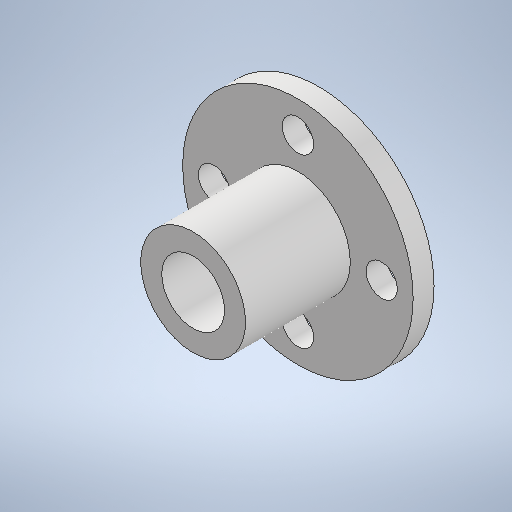
# Autodesk Inventor part: 驱动轮法兰
Saved by Autodesk Inventor 2025.1 (Build 291241000, 241)
## iProperties
Created: 2025-08-26
Part Number: 驱动轮法兰
Material: 常规
Document SubType Name: Modeling
Designer: Piw
Density: 1 g/cm^3
Appearance: 默认
Author: Piw
Autodesk Inventor part; units mm, degrees
ref_plane "YZ Plane" through (0, 0, 0) normal (1, 0, 0) x (0, 1, 0)
ref_plane "XZ Plane" through (0, 0, 0) normal (0, 1, 0) x (-1, 0, 0)
ref_plane "XY Plane" through (0, 0, 0) normal (0, 0, 1) x (1, 0, 0)
sketch "草图1" plane through (0, 0, 0) normal (0, 0, 1) x (1, 0, 0)
  circle A0 centre (0, 0) radius 11
  circle A1 centre (0, 0) radius 3
  dimension "d0" = 22
  dimension "d1" = 6
  constraints: 2 centre point, 2 coincident
  measures "d0" diameter of A0
  measures "d1" diameter of A1
extrude "拉伸1" add sketch "草图1" along normal blind 2
sketch "草图2" plane through (0, 0, 2) normal (0, 0, 1) x (1, 0, 0)
  circle A0 centre (0, 0) radius 3 projected
  circle A1 centre (0, 0) radius 5
  dimension "d4" = 10
  constraints: 1 centre point, 1 coincident
  measures "d4" diameter of A1
extrude "拉伸2" add sketch "草图2" along normal blind 10
sketch "草图3" plane through (0, 0, 2) normal (0, 0, 1) x (1, 0, 0)
  circle A0 centre (0, 0) radius 8 construction
  circle A1 centre (0, 8) radius 1.5
  line L0 (0, 16.5468) -> (0, -16.1007)
  circle A2 centre (-8, 0) radius 1.5
  circle A3 centre (0, -8) radius 1.5
  circle A4 centre (8, 0) radius 1.5
  dimension "d7" = 16
  dimension "d8" = 3
  dimension "d11" = 360
  constraints: 4 centre point, 2 end point, 2 vertical, 1 coincident, 1 point on line, 1 vertical alignment, 11 other
  measures "d8" diameter of A1
extrude "拉伸3" cut sketch "草图3" against normal blind 10
